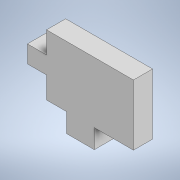
# Autodesk Inventor part: CotéV2
Saved by Autodesk Inventor 2020 (Build 240168000, 168)
## iProperties
Created: 2019-11-07
Part Number: CotéV2
Material: Générique
Document SubType Name: Modeling
Designer: erwan
Density: 1 g/cm^3
Appearance: Par défaut
Author: erwan
Autodesk Inventor part; units mm, degrees
ref_plane "YZ Plane" through (0, 0, 0) normal (1, 0, 0) x (0, 1, 0)
ref_plane "XZ Plane" through (0, 0, 0) normal (0, 1, 0) x (-1, 0, 0)
ref_plane "XY Plane" through (0, 0, 0) normal (0, 0, 1) x (1, 0, 0)
sketch "Esquisse1" plane through (0, 0, 0) normal (0, 1, 0) x (-1, 0, 0)
  line L0 (0, 0) -> (100, 0)
  line L1 (100, 0) -> (100, -22)
  line L2 (100, -22) -> (0, -22)
  line L3 (0, -22) -> (0, 0)
  dimension "d0" = 100
  dimension "d3" = 22
  constraints: 8 end point, 2 parallel, 1 horizontal, 1 perpendicular
  measures "d0" distance of L1.end L2.end
  measures "d3" distance of L2.end L0.start
extrude "Extrusion1" add sketch "Esquisse1" along normal blind 70
sketch "Esquisse2" plane through (-100, 0, 0) normal (0, 0, 1) x (1, 0, 0)
  line L0 (100, 0) -> (55, 0)
  line L1 (0, 0) -> (100, 0) projected
  line L2 (55, 0) -> (55, -22)
  line L3 (55, -22) -> (23, -22)
  line L4 (23, -22) -> (23, 0)
  line L5 (0, 70) -> (100, 70) projected
  line L6 (0, 70) -> (0, 45)
  line L7 (0, 0) -> (0, 70) projected
  line L8 (0, 45) -> (-22, 45)
  line L9 (-22, 45) -> (-22, 25)
  line L10 (-22, 25) -> (0, 25)
  dimension "d4" = 45
  dimension "d5" = 22
  dimension "d6" = 32
  dimension "d7" = 25
  dimension "d8" = 22
  dimension "d9" = 20
  constraints: 16 end point, 4 perpendicular, 4 point on line, 1 horizontal, 1 vertical
  measures "d4" distance of L0.start L0.end
  measures "d5" distance of L0.end L2.end
  measures "d6" distance of L2.end L3.end
  measures "d7" distance of L5.start L6.end
  measures "d8" distance of L6.end L8.end
  measures "d9" distance of L8.end L9.end
extrude "Extrusion2" add sketch "Esquisse2" against normal blind 22
